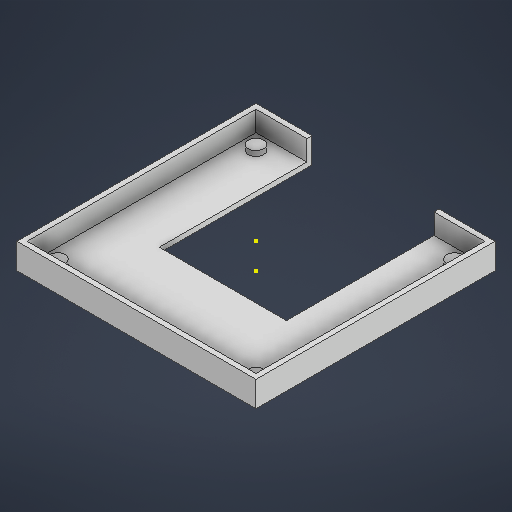
# Autodesk Inventor part: particle_sensor_case_bottom
Saved by Autodesk Inventor 2027 (Build 310192060, 192F)
## iProperties
Created: 2026-06-05
Part Number: particle_sensor_case_bottom
Material: Generic
Document SubType Name: Modeling
Designer: cmitchel
Density: 1 g/cm^3
Appearance: Default
Author: cmitchel
Autodesk Inventor part; units mm, degrees
ref_plane "YZ Plane" through (0, 0, 0) normal (1, 0, 0) x (0, 1, 0)
ref_plane "XZ Plane" through (0, 0, 0) normal (0, 1, 0) x (-1, 0, 0)
ref_plane "XY Plane" through (0, 0, 0) normal (0, 0, 1) x (1, 0, 0)
sketch "Sketch1" plane through (0, 0, 0) normal (0, 1, 0) x (-1, 0, 0)
  point P0 (0, 0)
sketch "Sketch2" plane through (0, 0, 0) normal (0, 1, 0) x (-1, 0, 0)
  line L0 (23.5, 23.5) -> (-23.5, 23.5)
  line L1 (-23.5, 23.5) -> (-23.5, -23.5)
  line L2 (-23.5, -23.5) -> (23.5, -23.5)
  line L3 (23.5, -23.5) -> (23.5, 23.5)
  point P0 (0, 0)
  dimension "d4" = 47
  dimension "d5" = 47
  dimension "d6" = 23.5
  dimension "d7" = 23.5
  constraints: 8 end point, 2 parallel, 1 horizontal, 1 perpendicular
  measures "d4" distance of L3.start L1.end
  measures "d5" distance of L3.start L3.end
  measures "d6" distance from line of point (0, 0) L2
  measures "d7" distance from line of point (0, 0) L3
extrude "Extrusion1" add sketch "Sketch2" along normal blind 5
sketch "Sketch3" plane through (0, 5, 0) normal (0, 1, 0) x (1, 0, 0)
  point P0 (0, 0)
sketch "Sketch4" plane through (0, 5, 0) normal (0, 1, 0) x (1, 0, 0)
  line L0 (-22.5, -22.5) -> (22.5, -22.5)
  line L1 (22.5, -22.5) -> (22.5, 22.5)
  line L2 (22.5, 22.5) -> (-22.5, 22.5)
  line L3 (-22.5, 22.5) -> (-22.5, -22.5)
  point P0 (0, 0)
  dimension "d10" = 45
  dimension "d11" = 45
  dimension "d12" = 22.5
  dimension "d13" = 22.5
  constraints: 8 end point, 2 parallel, 1 horizontal, 1 perpendicular
  measures "d10" distance between parallel lines of L1 L3
  measures "d11" distance of L0.end L1.end
  measures "d12" distance from line of point (0, 0) L2
  measures "d13" distance from line of point (0, 0) L3
extrude "Extrusion2" cut sketch "Sketch4" against normal blind 4
sketch "Sketch5" plane through (0, 5, 0) normal (0, 1, 0) x (1, 0, 0)
  line L0 (23.5, 23.5) -> (-23.5, 23.5) projected
  line L1 (12.5, 23.5) -> (-12.5, 23.5)
  line L2 (-12.5, 23.5) -> (-12.5, -6.5)
  line L3 (-12.5, -6.5) -> (12.5, -6.5)
  line L4 (12.5, -6.5) -> (12.5, 23.5)
  point P0 (0, 0)
  dimension "d16" = 30
  dimension "d17" = 25
  dimension "d18" = 12.5
  constraints: 8 end point, 2 parallel, 1 horizontal, 1 perpendicular, 1 point on line
  measures "d16" distance of L1.end L2.end
  measures "d17" distance of L2.end L3.end
  measures "d18" distance from line of point (0, 0) L2
extrude "Extrusion3" cut sketch "Sketch5" against normal blind 10
sketch "Sketch6" plane through (0, 1, 0) normal (0, 1, 0) x (1, 0, 0)
  circle A0 centre (-19.5, -19.5) radius 1.5
  line L0 (-23.5, 23.5) -> (-23.5, -23.5) projected
  line L1 (-23.5, -23.5) -> (23.5, -23.5) projected
  line L2 (0, 0) -> (-11.992, 0) construction
  line L3 (0, 0) -> (0, -9.7427) construction
  circle A1 centre (-19.5, 19.5) radius 1.5
  line L4 (-22.5, -22.5) -> (-22.5, 22.5) projected
  line L5 (22.5, -22.5) -> (-22.5, -22.5) projected
  circle A2 centre (19.5, -19.5) radius 1.5
  circle A3 centre (19.5, 19.5) radius 1.5
  dimension "d21" = 3
  dimension "d24" = 3
  dimension "d25" = 3
  dimension "d26" = 3
  dimension "d27" = 3
  dimension "d28" = 3
  constraints: 4 centre point, 4 end point, 3 symmetric about line, 1 horizontal, 1 vertical
  measures "d21" diameter of A0
  measures "d24" diameter of A1
  measures "d25" distance from line of L4 A0.centre
  measures "d26" distance from line of L5 A0.centre
  measures "d27" diameter of A2
  measures "d28" diameter of A3
extrude "Extrusion4" add sketch "Sketch6" along normal blind 1
body "Solid1"
